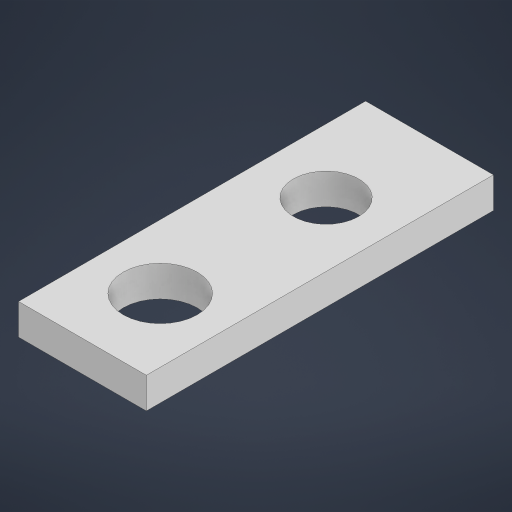
# Autodesk Inventor part: da
Saved by Autodesk Inventor 2024.3 (Build 283343000, 343)
## iProperties
Created: 2025-06-22
Part Number: da
Material: Generic
Document SubType Name: Modeling
Designer: Akbar Syihabuddin
Density: 1 g/cm^3
Appearance: Default
Author: Akbar Syihabuddin
Autodesk Inventor part; units mm, degrees
ref_plane "YZ Plane" through (0, 0, 0) normal (1, 0, 0) x (0, 1, 0)
ref_plane "XZ Plane" through (0, 0, 0) normal (0, 1, 0) x (-1, 0, 0)
ref_plane "XY Plane" through (0, 0, 0) normal (0, 0, 1) x (1, 0, 0)
sketch "Sketch1" plane through (0, 0, 0) normal (0, 1, 0) x (-1, 0, 0)
  line L0 (-5.8441, 11.034) -> (2.4286, 11.034)
  line L1 (2.4286, 11.034) -> (2.4286, -11.4332)
  line L2 (2.4286, -11.4332) -> (-5.8441, -11.4332)
  line L3 (-5.8441, -11.4332) -> (-5.8441, 11.034)
  circle A0 centre (-1.7078, 5.9994) radius 2.3953
  circle A1 centre (-1.7078, -4.7352) radius 2.113
  point P0 (0, 0)
  constraints: 8 end point, 2 centre point, 2 parallel, 1 horizontal, 1 perpendicular
extrude "Extrusion1" add sketch "Sketch1" along normal blind 2
body "Solid1"
